Autodesk Fusion 360 part; units mm, degrees
(part 7 of 7)
  line L506 (59.905, -71.6419) -> (59.8713, -71.7229)
  line L507 (59.8713, -71.7229) -> (59.8391, -71.8051)
  line L508 (59.8391, -71.8051) -> (59.9395, -71.9042)
  line L509 (59.9395, -71.9042) -> (60.0412, -72.002)
  line L510 (60.0412, -72.002) -> (60.1441, -72.0986)
  line L511 (60.1441, -72.0986) -> (60.225, -72.0631)
  line L512 (60.225, -72.0631) -> (60.3047, -72.0264)
  line L513 (60.3047, -72.0264) -> (60.3829, -71.9882)
  line L514 (60.3829, -71.9882) -> (60.4597, -71.9486)
  line L515 (60.4597, -71.9486) -> (60.535, -71.9075)
  line L516 (60.535, -71.9075) -> (60.6087, -71.8648)
  line L517 (60.6087, -71.8648) -> (60.6807, -71.8206)
  line L518 (60.6807, -71.8206) -> (60.7508, -71.7746)
  line L519 (60.7508, -71.7746) -> (60.8189, -71.7268)
  line L520 (60.8189, -71.7268) -> (60.8846, -71.6768)
  line L521 (60.8846, -71.6768) -> (60.9474, -71.6243)
  line L522 (60.9474, -71.6243) -> (61.006, -71.568)
  line L523 (61.006, -71.568) -> (61.2294, -71.3134)
  line L524 (61.2294, -71.3134) -> (61.3835, -71.4459)
  line L525 (61.3835, -71.4459) -> (61.5404, -71.5752)
  line L526 (61.5404, -71.5752) -> (61.7, -71.7012)
  line L527 (61.7, -71.7012) -> (61.8621, -71.8238)
  line L528 (61.8621, -71.8238) -> (61.6605, -72.096)
  line L529 (61.6605, -72.096) -> (61.6179, -72.1651)
  line L530 (61.6179, -72.1651) -> (61.5798, -72.2377)
  line L531 (61.5798, -72.2377) -> (61.5449, -72.3125)
  line L532 (61.5449, -72.3125) -> (61.5125, -72.3891)
  line L533 (61.5125, -72.3891) -> (61.4824, -72.4674)
  line L534 (61.4824, -72.4674) -> (61.4544, -72.5471)
  line L535 (61.4544, -72.5471) -> (61.4283, -72.6281)
  line L536 (61.4283, -72.6281) -> (61.4041, -72.7104)
  line L537 (61.4041, -72.7104) -> (61.3816, -72.7939)
  line L538 (61.3816, -72.7939) -> (61.3609, -72.8784)
  line L539 (61.3609, -72.8784) -> (61.3418, -72.964)
  line L540 (61.3418, -72.964) -> (61.3242, -73.0507)
  line L541 (61.3242, -73.0507) -> (61.4404, -73.1308)
  line L542 (61.4404, -73.1308) -> (61.5575, -73.2095)
  line L543 (61.5575, -73.2095) -> (61.6756, -73.2867)
  line L544 (61.6756, -73.2867) -> (61.7492, -73.2378)
  line L545 (61.7492, -73.2378) -> (61.8212, -73.1877)
  line L546 (61.8212, -73.1877) -> (61.8916, -73.1365)
  line L547 (61.8916, -73.1365) -> (61.9604, -73.0841)
  line L548 (61.9604, -73.0841) -> (62.0274, -73.0306)
  line L549 (62.0274, -73.0306) -> (62.0926, -72.9758)
  line L550 (62.0926, -72.9758) -> (62.1558, -72.9198)
  line L551 (62.1558, -72.9198) -> (62.2169, -72.8623)
  line L552 (62.2169, -72.8623) -> (62.2756, -72.8034)
  line L553 (62.2756, -72.8034) -> (62.3316, -72.7427)
  line L554 (62.3316, -72.7427) -> (62.3844, -72.6801)
  line L555 (62.3844, -72.6801) -> (62.4323, -72.6145)
  line L556 (62.4323, -72.6145) -> (62.608, -72.325)
  line L557 (62.608, -72.325) -> (62.7829, -72.4287)
  line L558 (62.7829, -72.4287) -> (62.9599, -72.5288)
  line L559 (62.9599, -72.5288) -> (63.1388, -72.6252)
  line L560 (63.1388, -72.6252) -> (63.3198, -72.7178)
  line L561 (63.3198, -72.7178) -> (63.1686, -73.0209)
  line L562 (63.1686, -73.0209) -> (63.1386, -73.0963)
  line L563 (63.1386, -73.0963) -> (63.1137, -73.1744)
  line L564 (63.1137, -73.1744) -> (63.0923, -73.2541)
  line L565 (63.0923, -73.2541) -> (63.0737, -73.3352)
  line L566 (63.0737, -73.3352) -> (63.0577, -73.4175)
  line L567 (63.0577, -73.4175) -> (63.0439, -73.5009)
  line L568 (63.0439, -73.5009) -> (63.0323, -73.5852)
  line L569 (63.0323, -73.5852) -> (63.0227, -73.6704)
  line L570 (63.0227, -73.6704) -> (63.0151, -73.7565)
  line L571 (63.0151, -73.7565) -> (63.0093, -73.8434)
  line L572 (63.0093, -73.8434) -> (63.0054, -73.9311)
  line L573 (63.0054, -73.9311) -> (63.0032, -74.0194)
  line L574 (63.0032, -74.0194) -> (63.1314, -74.0782)
  line L575 (63.1314, -74.0782) -> (63.2604, -74.1353)
  line L576 (63.2604, -74.1353) -> (63.3901, -74.1908)
  line L577 (63.3901, -74.1908) -> (63.4541, -74.1299)
  line L578 (63.4541, -74.1299) -> (63.5163, -74.068)
  line L579 (63.5163, -74.068) -> (63.5768, -74.0054)
  line L580 (63.5768, -74.0054) -> (63.6355, -73.9419)
  line L581 (63.6355, -73.9419) -> (63.6922, -73.8775)
  line L582 (63.6922, -73.8775) -> (63.7468, -73.8123)
  line L583 (63.7468, -73.8123) -> (63.7993, -73.7461)
  line L584 (63.7993, -73.7461) -> (63.8495, -73.6789)
  line L585 (63.8495, -73.6789) -> (63.8971, -73.6106)
  line L586 (63.8971, -73.6106) -> (63.9418, -73.5412)
  line L587 (63.9418, -73.5412) -> (63.9829, -73.4704)
  line L588 (63.9829, -73.4704) -> (64.0186, -73.3974)
  line L589 (64.0186, -73.3974) -> (64.1414, -73.0818)
  line L590 (64.1414, -73.0818) -> (64.3316, -73.1536)
  line L591 (64.3316, -73.1536) -> (64.5233, -73.2214)
  line L592 (64.5233, -73.2214) -> (64.7163, -73.2852)
  line L593 (64.7163, -73.2852) -> (64.9106, -73.3451)
  line L594 (64.9106, -73.3451) -> (64.8143, -73.6698)
  line L595 (64.8143, -73.6698) -> (64.7978, -73.7493)
  line L596 (64.7978, -73.7493) -> (64.7869, -73.8305)
  line L597 (64.7869, -73.8305) -> (64.7797, -73.9127)
  line L598 (64.7797, -73.9127) -> (64.7755, -73.9958)
  line L599 (64.7755, -73.9958) -> (64.7739, -74.0796)
  line L600 (64.7739, -74.0796) -> (64.7749, -74.1641)
  line L601 (64.7749, -74.1641) -> (64.7781, -74.2492)
  line L602 (64.7781, -74.2492) -> (64.7835, -74.3348)
  line L603 (64.7835, -74.3348) -> (64.7909, -74.4209)
  line L604 (64.7909, -74.4209) -> (64.8003, -74.5075)
  line L605 (64.8003, -74.5075) -> (64.8116, -74.5945)
  line L606 (64.8116, -74.5945) -> (64.8248, -74.6819)
  line L607 (64.8248, -74.6819) -> (64.9613, -74.7175)
  line L608 (64.9613, -74.7175) -> (65.0983, -74.7514)
  line L609 (65.0983, -74.7514) -> (65.2357, -74.7835)
  line L610 (65.2357, -74.7835) -> (65.2881, -74.7123)
  line L611 (65.2881, -74.7123) -> (65.3386, -74.6407)
  line L612 (65.3386, -74.6407) -> (65.3873, -74.5685)
  line L613 (65.3873, -74.5685) -> (65.434, -74.4957)
  line L614 (65.434, -74.4957) -> (65.4787, -74.4225)
  line L615 (65.4787, -74.4225) -> (65.5212, -74.3487)
  line L616 (65.5212, -74.3487) -> (65.5614, -74.2744)
  line L617 (65.5614, -74.2744) -> (65.5991, -74.1996)
  line L618 (65.5991, -74.1996) -> (65.6342, -74.1241)
  line L619 (65.6342, -74.1241) -> (65.6661, -74.048)
  line L620 (65.6661, -74.048) -> (65.6943, -73.9711)
  line L621 (65.6943, -73.9711) -> (65.7168, -73.893)
  line L622 (65.7168, -73.893) -> (65.783, -73.5609)
  line L623 (65.783, -73.5609) -> (65.9827, -73.5985)
  line L624 (65.9827, -73.5985) -> (66.1833, -73.632)
  line L625 (66.1833, -73.632) -> (66.3844, -73.6614)
  line L626 (66.3844, -73.6614) -> (66.5861, -73.6866)
  line L627 (66.5861, -73.6866) -> (66.5477, -74.023)
  line L628 (66.5477, -74.023) -> (66.5453, -74.1042)
  line L629 (66.5453, -74.1042) -> (66.5486, -74.1861)
  line L630 (66.5486, -74.1861) -> (66.5558, -74.2683)
  line L631 (66.5558, -74.2683) -> (66.5661, -74.3509)
  line L632 (66.5661, -74.3509) -> (66.5791, -74.4337)
  line L633 (66.5791, -74.4337) -> (66.5947, -74.5167)
  line L634 (66.5947, -74.5167) -> (66.6126, -74.6)
  line L635 (66.6126, -74.6) -> (66.6328, -74.6834)
  line L636 (66.6328, -74.6834) -> (66.6551, -74.7669)
  line L637 (66.6551, -74.7669) -> (66.6794, -74.8505)
  line L638 (66.6794, -74.8505) -> (66.7056, -74.9342)
  line L639 (66.7056, -74.9342) -> (66.7338, -75.0179)
  line L640 (66.7338, -75.0179) -> (66.8744, -75.0293)
  line L641 (66.8744, -75.0293) -> (67.0152, -75.0389)
  line L642 (67.0152, -75.0389) -> (67.1561, -75.0467)
  line L643 (67.1561, -75.0467) -> (67.1953, -74.9675)
  line L644 (67.1953, -74.9675) -> (67.2326, -74.8881)
  line L645 (67.2326, -74.8881) -> (67.268, -74.8086)
  line L646 (67.268, -74.8086) -> (67.3014, -74.7289)
  line L647 (67.3014, -74.7289) -> (67.3327, -74.649)
  line L648 (67.3327, -74.649) -> (67.3618, -74.569)
  line L649 (67.3618, -74.569) -> (67.3884, -74.4888)
  line L650 (67.3884, -74.4888) -> (67.4126, -74.4085)
  line L651 (67.4126, -74.4085) -> (67.434, -74.3281)
  line L652 (67.434, -74.3281) -> (67.4522, -74.2476)
  line L653 (67.4522, -74.2476) -> (67.4666, -74.167)
  line L654 (67.4666, -74.167) -> (67.4752, -74.0862)
  line L655 (67.4752, -74.0862) -> (67.4827, -73.7476)
  line L656 (67.4827, -73.7476) -> (67.686, -73.75)
  line L657 (67.686, -73.75) -> (67.8893, -73.7482)
  line L658 (67.8893, -73.7482) -> (68.0925, -73.7421)
  line L659 (68.0925, -73.7421) -> (68.2955, -73.7319)
  line L660 (68.2955, -73.7319) -> (68.3161, -74.07)
  line L661 (68.3161, -74.07) -> (68.3278, -74.1503)
  line L662 (68.3278, -74.1503) -> (68.3453, -74.2304)
  line L663 (68.3453, -74.2304) -> (68.3666, -74.3101)
  line L664 (68.3666, -74.3101) -> (68.3911, -74.3896)
  line L665 (68.3911, -74.3896) -> (68.4184, -74.4689)
  line L666 (68.4184, -74.4689) -> (68.4481, -74.548)
  line L667 (68.4481, -74.548) -> (68.4803, -74.6268)
  line L668 (68.4803, -74.6268) -> (68.5146, -74.7055)
  line L669 (68.5146, -74.7055) -> (68.551, -74.7838)
  line L670 (68.551, -74.7838) -> (68.5895, -74.862)
  line L671 (68.5895, -74.862) -> (68.6298, -74.9398)
  line L672 (68.6298, -74.9398) -> (68.6721, -75.0174)
  line L673 (68.6721, -75.0174) -> (68.8126, -75.0042)
  line L674 (68.8126, -75.0042) -> (68.9529, -74.9892)
  line L675 (68.9529, -74.9892) -> (69.093, -74.9724)
  line L676 (69.093, -74.9724) -> (69.1179, -74.8876)
  line L677 (69.1179, -74.8876) -> (69.1409, -74.803)
  line L678 (69.1409, -74.803) -> (69.1619, -74.7185)
  line L679 (69.1619, -74.7185) -> (69.181, -74.6342)
  line L680 (69.181, -74.6342) -> (69.1979, -74.5501)
  line L681 (69.1979, -74.5501) -> (69.2126, -74.4662)
  line L682 (69.2126, -74.4662) -> (69.225, -74.3826)
  line L683 (69.225, -74.3826) -> (69.2348, -74.2994)
  line L684 (69.2348, -74.2994) -> (69.2419, -74.2165)
  line L685 (69.2419, -74.2165) -> (69.2459, -74.134)
  line L686 (69.2459, -74.134) -> (69.246, -74.0521)
  line L687 (69.246, -74.0521) -> (69.2405, -73.9711)
  line L688 (69.2405, -73.9711) -> (69.1891, -73.6363)
  line L689 (69.1891, -73.6363) -> (69.3897, -73.6034)
  line L690 (69.3897, -73.6034) -> (69.5896, -73.5663)
  line L691 (69.5896, -73.5663) -> (69.7887, -73.5251)
  line L692 (69.7887, -73.5251) -> (69.9868, -73.4797)
  line L693 (69.9868, -73.4797) -> (70.0658, -73.8091)
  line L694 (70.0658, -73.8091) -> (70.0913, -73.8862)
  line L695 (70.0913, -73.8862) -> (70.1224, -73.962)
  line L696 (70.1224, -73.962) -> (70.1573, -74.0368)
  line L697 (70.1573, -74.0368) -> (70.1952, -74.1109)
  line L698 (70.1952, -74.1109) -> (70.2358, -74.1842)
  line L699 (70.2358, -74.1842) -> (70.2788, -74.2569)
  line L700 (70.2788, -74.2569) -> (70.3241, -74.329)
  line L701 (70.3241, -74.329) -> (70.3716, -74.4005)
  line L702 (70.3716, -74.4005) -> (70.4211, -74.4713)
  line L703 (70.4211, -74.4713) -> (70.4725, -74.5416)
  line L704 (70.4725, -74.5416) -> (70.5258, -74.6112)
  line L705 (70.5258, -74.6112) -> (70.5809, -74.6803)
  line L706 (70.5809, -74.6803) -> (70.717, -74.6429)
  line L707 (70.717, -74.6429) -> (70.8525, -74.6038)
  line L708 (70.8525, -74.6038) -> (70.9876, -74.5629)
  line L709 (70.9876, -74.5629) -> (70.9974, -74.4751)
  line L710 (70.9974, -74.4751) -> (71.0053, -74.3877)
  line L711 (71.0053, -74.3877) -> (71.0114, -74.3009)
  line L712 (71.0114, -74.3009) -> (71.0155, -74.2145)
  line L713 (71.0155, -74.2145) -> (71.0175, -74.1288)
  line L714 (71.0175, -74.1288) -> (71.0175, -74.0436)
  line L715 (71.0175, -74.0436) -> (71.0151, -73.9592)
  line L716 (71.0151, -73.9592) -> (71.0104, -73.8755)
  line L717 (71.0104, -73.8755) -> (71.003, -73.7926)
  line L718 (71.003, -73.7926) -> (70.9926, -73.7107)
  line L719 (70.9926, -73.7107) -> (70.9785, -73.63)
  line L720 (70.9785, -73.63) -> (70.959, -73.5512)
  line L721 (70.959, -73.5512) -> (70.8502, -73.2304)
  line L722 (70.8502, -73.2304) -> (71.0421, -73.1632)
  line L723 (71.0421, -73.1632) -> (71.2325, -73.0919)
  line L724 (71.2325, -73.0919) -> (71.4214, -73.0168)
  line L725 (71.4214, -73.0168) -> (71.6087, -72.9377)
  line L726 (71.6087, -72.9377) -> (71.7436, -73.2483)
  line L727 (71.7436, -73.2483) -> (71.7821, -73.3198)
  line L728 (71.7821, -73.3198) -> (71.8259, -73.389)
  line L729 (71.8259, -73.389) -> (71.8732, -73.4567)
  line L730 (71.8732, -73.4567) -> (71.9234, -73.5231)
  line L731 (71.9234, -73.5231) -> (71.9761, -73.5883)
  line L732 (71.9761, -73.5883) -> (72.0312, -73.6524)
  line L733 (72.0312, -73.6524) -> (72.0883, -73.7155)
  line L734 (72.0883, -73.7155) -> (72.1475, -73.7776)
  line L735 (72.1475, -73.7776) -> (72.2085, -73.8388)
  line L736 (72.2085, -73.8388) -> (72.2713, -73.8991)
  line L737 (72.2713, -73.8991) -> (72.3359, -73.9584)
  line L738 (72.3359, -73.9584) -> (72.4022, -74.0169)
  line L739 (72.4022, -74.0169) -> (72.5297, -73.9564)
  line L740 (72.5297, -73.9564) -> (72.6564, -73.8943)
  line L741 (72.6564, -73.8943) -> (72.7823, -73.8306)
  line L742 (72.7823, -73.8306) -> (72.7767, -73.7425)
  line L743 (72.7767, -73.7425) -> (72.7693, -73.655)
  line L744 (72.7693, -73.655) -> (72.7602, -73.5685)
  line L745 (72.7602, -73.5685) -> (72.7493, -73.4827)
  line L746 (72.7493, -73.4827) -> (72.7364, -73.3979)
  line L747 (72.7364, -73.3979) -> (72.7215, -73.3141)
  line L748 (72.7215, -73.3141) -> (72.7046, -73.2313)
  line L749 (72.7046, -73.2313) -> (72.6854, -73.1497)
  line L750 (72.6854, -73.1497) -> (72.6637, -73.0694)
  line L751 (72.6637, -73.0694) -> (72.6392, -72.9905)
  line L752 (72.6392, -72.9905) -> (72.6114, -72.9135)
  line L753 (72.6114, -72.9135) -> (72.5784, -72.8392)
  line L754 (72.5784, -72.8392) -> (72.4156, -72.5423)
  line L755 (72.4156, -72.5423) -> (72.5929, -72.4427)
  line L756 (72.5929, -72.4427) -> (72.768, -72.3395)
  line L757 (72.768, -72.3395) -> (72.941, -72.2327)
  line L758 (72.941, -72.2327) -> (73.1117, -72.1223)
  line L759 (73.1117, -72.1223) -> (73.2985, -72.4048)
  line L760 (73.2985, -72.4048) -> (73.3489, -72.4685)
  line L761 (73.3489, -72.4685) -> (73.4041, -72.529)
  line L762 (73.4041, -72.529) -> (73.4624, -72.5874)
  line L763 (73.4624, -72.5874) -> (73.5233, -72.6441)
  line L764 (73.5233, -72.6441) -> (73.5866, -72.6991)
  line L765 (73.5866, -72.6991) -> (73.6519, -72.7527)
  line L766 (73.6519, -72.7527) -> (73.7191, -72.8049)
  line L767 (73.7191, -72.8049) -> (73.7882, -72.8559)
  line L768 (73.7882, -72.8559) -> (73.8589, -72.9055)
  line L769 (73.8589, -72.9055) -> (73.9313, -72.954)
  line L770 (73.9313, -72.954) -> (74.0052, -73.0012)
  line L771 (74.0052, -73.0012) -> (74.0806, -73.0473)
  line L772 (74.0806, -73.0473) -> (74.1956, -72.9656)
  line L773 (74.1956, -72.9656) -> (74.3096, -72.8824)
  line L774 (74.3096, -72.8824) -> (74.4226, -72.7979)
  line L775 (74.4226, -72.7979) -> (74.4017, -72.712)
  line L776 (74.4017, -72.712) -> (74.3793, -72.6272)
  line L777 (74.3793, -72.6272) -> (74.3553, -72.5435)
  line L778 (74.3553, -72.5435) -> (74.3296, -72.4609)
  line L779 (74.3296, -72.4609) -> (74.3022, -72.3797)
  line L780 (74.3022, -72.3797) -> (74.273, -72.2997)
  line L781 (74.273, -72.2997) -> (74.242, -72.2211)
  line L782 (74.242, -72.2211) -> (74.2089, -72.1441)
  line L783 (74.2089, -72.1441) -> (74.1736, -72.0687)
  line L784 (74.1736, -72.0687) -> (74.1358, -71.9953)
  line L785 (74.1358, -71.9953) -> (74.095, -71.9243)
  line L786 (74.095, -71.9243) -> (74.0497, -71.8569)
  line L787 (74.0497, -71.8569) -> (73.8378, -71.5927)
  line L788 (73.8378, -71.5927) -> (73.995, -71.4639)
  line L789 (73.995, -71.4639) -> (74.1496, -71.3318)
  line L790 (74.1496, -71.3318) -> (74.3014, -71.1966)
  line L791 (74.3014, -71.1966) -> (74.4503, -71.0582)
  line L792 (74.4503, -71.0582) -> (74.6834, -71.304)
  line L793 (74.6834, -71.304) -> (74.744, -71.358)
  line L794 (74.744, -71.358) -> (74.8089, -71.4081)
  line L795 (74.8089, -71.4081) -> (74.8765, -71.4554)
  line L796 (74.8765, -71.4554) -> (74.9463, -71.5006)
  line L797 (74.9463, -71.5006) -> (75.0182, -71.5439)
  line L798 (75.0182, -71.5439) -> (75.0918, -71.5853)
  line L799 (75.0918, -71.5853) -> (75.1671, -71.6251)
  line L800 (75.1671, -71.6251) -> (75.2439, -71.6632)
  line L801 (75.2439, -71.6632) -> (75.3222, -71.6998)
  line L802 (75.3222, -71.6998) -> (75.4019, -71.735)
  line L803 (75.4019, -71.735) -> (75.4829, -71.7687)
  line L804 (75.4829, -71.7687) -> (75.5651, -71.8009)
  line L805 (75.5651, -71.8009) -> (75.6642, -71.7005)
  line L806 (75.6642, -71.7005) -> (75.762, -71.5988)
  line L807 (75.762, -71.5988) -> (75.8586, -71.4959)
  line L808 (75.8586, -71.4959) -> (75.8231, -71.415)
  line L809 (75.8231, -71.415) -> (75.7864, -71.3353)
  line L810 (75.7864, -71.3353) -> (75.7482, -71.2571)
  line L811 (75.7482, -71.2571) -> (75.7086, -71.1803)
  line L812 (75.7086, -71.1803) -> (75.6675, -71.105)
  line L813 (75.6675, -71.105) -> (75.6248, -71.0313)
  line L814 (75.6248, -71.0313) -> (75.5806, -70.9593)
  line L815 (75.5806, -70.9593) -> (75.5346, -70.8892)
  line L816 (75.5346, -70.8892) -> (75.4868, -70.8211)
  line L817 (75.4868, -70.8211) -> (75.4368, -70.7554)
  line L818 (75.4368, -70.7554) -> (75.3843, -70.6926)
  line L819 (75.3843, -70.6926) -> (75.328, -70.634)
  line L820 (75.328, -70.634) -> (75.0734, -70.4106)
  line L821 (75.0734, -70.4106) -> (75.2059, -70.2565)
  line L822 (75.2059, -70.2565) -> (75.3352, -70.0996)
  line L823 (75.3352, -70.0996) -> (75.4612, -69.94)
  line L824 (75.4612, -69.94) -> (75.5838, -69.7779)
  line L825 (75.5838, -69.7779) -> (75.856, -69.9795)
  line L826 (75.856, -69.9795) -> (75.9251, -70.0221)
  line L827 (75.9251, -70.0221) -> (75.9977, -70.0602)
  line L828 (75.9977, -70.0602) -> (76.0725, -70.0951)
  line L829 (76.0725, -70.0951) -> (76.1491, -70.1275)
  line L830 (76.1491, -70.1275) -> (76.2274, -70.1576)
  line L831 (76.2274, -70.1576) -> (76.3071, -70.1856)
  line L832 (76.3071, -70.1856) -> (76.3881, -70.2117)
  line L833 (76.3881, -70.2117) -> (76.4704, -70.2359)
  line L834 (76.4704, -70.2359) -> (76.5539, -70.2584)
  line L835 (76.5539, -70.2584) -> (76.6384, -70.2791)
  line L836 (76.6384, -70.2791) -> (76.724, -70.2982)
  line L837 (76.724, -70.2982) -> (76.8107, -70.3158)
  line L838 (76.8107, -70.3158) -> (76.8908, -70.1996)
  line L839 (76.8908, -70.1996) -> (76.9695, -70.0825)
  line L840 (76.9695, -70.0825) -> (77.0467, -69.9644)
  line L841 (77.0467, -69.9644) -> (76.9978, -69.8908)
  line L842 (76.9978, -69.8908) -> (76.9477, -69.8188)
  line L843 (76.9477, -69.8188) -> (76.8965, -69.7484)
  line L844 (76.8965, -69.7484) -> (76.8441, -69.6796)
  line L845 (76.8441, -69.6796) -> (76.7906, -69.6126)
  line L846 (76.7906, -69.6126) -> (76.7358, -69.5474)
  line L847 (76.7358, -69.5474) -> (76.6798, -69.4842)
  line L848 (76.6798, -69.4842) -> (76.6223, -69.4231)
  line L849 (76.6223, -69.4231) -> (76.5634, -69.3644)
  line L850 (76.5634, -69.3644) -> (76.5027, -69.3084)
  line L851 (76.5027, -69.3084) -> (76.4401, -69.2556)
  line L852 (76.4401, -69.2556) -> (76.3745, -69.2077)
  line L853 (76.3745, -69.2077) -> (76.085, -69.032)
  line L854 (76.085, -69.032) -> (76.1887, -68.8571)
  line L855 (76.1887, -68.8571) -> (76.2888, -68.6801)
  line L856 (76.2888, -68.6801) -> (76.3852, -68.5012)
  line L857 (76.3852, -68.5012) -> (76.4778, -68.3202)
  line L858 (76.4778, -68.3202) -> (76.7809, -68.4714)
  line L859 (76.7809, -68.4714) -> (76.8563, -68.5014)
  line L860 (76.8563, -68.5014) -> (76.9344, -68.5263)
  line L861 (76.9344, -68.5263) -> (77.0141, -68.5477)
  line L862 (77.0141, -68.5477) -> (77.0952, -68.5663)
  line L863 (77.0952, -68.5663) -> (77.1775, -68.5823)
  line L864 (77.1775, -68.5823) -> (77.2609, -68.5961)
  line L865 (77.2609, -68.5961) -> (77.3452, -68.6077)
  line L866 (77.3452, -68.6077) -> (77.4304, -68.6173)
  line L867 (77.4304, -68.6173) -> (77.5165, -68.6249)
  line L868 (77.5165, -68.6249) -> (77.6034, -68.6307)
  line L869 (77.6034, -68.6307) -> (77.6911, -68.6346)
  line L870 (77.6911, -68.6346) -> (77.7794, -68.6368)
  line L871 (77.7794, -68.6368) -> (77.8382, -68.5086)
  line L872 (77.8382, -68.5086) -> (77.8953, -68.3796)
  line L873 (77.8953, -68.3796) -> (77.9508, -68.2499)
  line L874 (77.9508, -68.2499) -> (77.8899, -68.1859)
  line L875 (77.8899, -68.1859) -> (77.828, -68.1237)
  line L876 (77.828, -68.1237) -> (77.7654, -68.0632)
  line L877 (77.7654, -68.0632) -> (77.7019, -68.0045)
  line L878 (77.7019, -68.0045) -> (77.6375, -67.9478)
  line L879 (77.6375, -67.9478) -> (77.5723, -67.8932)
  line L880 (77.5723, -67.8932) -> (77.5061, -67.8407)
  line L881 (77.5061, -67.8407) -> (77.4389, -67.7905)
  line L882 (77.4389, -67.7905) -> (77.3706, -67.7429)
  line L883 (77.3706, -67.7429) -> (77.3012, -67.6982)
  line L884 (77.3012, -67.6982) -> (77.2304, -67.6571)
  line L885 (77.2304, -67.6571) -> (77.1574, -67.6214)
  line L886 (77.1574, -67.6214) -> (76.8418, -67.4986)
  line L887 (76.8418, -67.4986) -> (76.9136, -67.3084)
  line L888 (76.9136, -67.3084) -> (76.9814, -67.1167)
  line L889 (76.9814, -67.1167) -> (77.0452, -66.9237)
  line L890 (77.0452, -66.9237) -> (77.1051, -66.7294)
  line L891 (77.1051, -66.7294) -> (77.4298, -66.8257)
  line L892 (77.4298, -66.8257) -> (77.5093, -66.8422)
  line L893 (77.5093, -66.8422) -> (77.5905, -66.8531)
  line L894 (77.5905, -66.8531) -> (77.6727, -66.8603)
  line L895 (77.6727, -66.8603) -> (77.7558, -66.8645)
  line L896 (77.7558, -66.8645) -> (77.8396, -66.8661)
  line L897 (77.8396, -66.8661) -> (77.9241, -66.8651)
  line L898 (77.9241, -66.8651) -> (78.0092, -66.8619)
  line L899 (78.0092, -66.8619) -> (78.0948, -66.8565)
  line L900 (78.0948, -66.8565) -> (78.1809, -66.8491)
  line L901 (78.1809, -66.8491) -> (78.2675, -66.8397)
  line L902 (78.2675, -66.8397) -> (78.3545, -66.8284)
  line L903 (78.3545, -66.8284) -> (78.4419, -66.8152)
  line L904 (78.4419, -66.8152) -> (78.4775, -66.6787)
  line L905 (78.4775, -66.6787) -> (78.5114, -66.5417)
  line L906 (78.5114, -66.5417) -> (78.5435, -66.4043)
  line L907 (78.5435, -66.4043) -> (78.4723, -66.3519)
  line L908 (78.4723, -66.3519) -> (78.4007, -66.3014)
  line L909 (78.4007, -66.3014) -> (78.3285, -66.2527)
  line L910 (78.3285, -66.2527) -> (78.2557, -66.206)
  line L911 (78.2557, -66.206) -> (78.1825, -66.1613)
  line L912 (78.1825, -66.1613) -> (78.1087, -66.1188)
  line L913 (78.1087, -66.1188) -> (78.0344, -66.0786)
  line L914 (78.0344, -66.0786) -> (77.9596, -66.0409)
  line L915 (77.9596, -66.0409) -> (77.8841, -66.0058)
  line L916 (77.8841, -66.0058) -> (77.808, -65.9739)
  line L917 (77.808, -65.9739) -> (77.7311, -65.9457)
  line L918 (77.7311, -65.9457) -> (77.653, -65.9232)
  line L919 (77.653, -65.9232) -> (77.3209, -65.857)
  line L920 (77.3209, -65.857) -> (77.3585, -65.6573)
  line L921 (77.3585, -65.6573) -> (77.392, -65.4567)
  line L922 (77.392, -65.4567) -> (77.4214, -65.2556)
  line L923 (77.4214, -65.2556) -> (77.4466, -65.0539)
  line L924 (77.4466, -65.0539) -> (77.783, -65.0923)
  line L925 (77.783, -65.0923) -> (77.8642, -65.0947)
  line L926 (77.8642, -65.0947) -> (77.9461, -65.0914)
  line L927 (77.9461, -65.0914) -> (78.0283, -65.0842)
  line L928 (78.0283, -65.0842) -> (78.1109, -65.0739)
  line L929 (78.1109, -65.0739) -> (78.1937, -65.0609)
  line L930 (78.1937, -65.0609) -> (78.2767, -65.0453)
  line L931 (78.2767, -65.0453) -> (78.36, -65.0274)
  line L932 (78.36, -65.0274) -> (78.4434, -65.0072)
  line L933 (78.4434, -65.0072) -> (78.5269, -64.9849)
  line L934 (78.5269, -64.9849) -> (78.6105, -64.9606)
  line L935 (78.6105, -64.9606) -> (78.6942, -64.9344)
  line L936 (78.6942, -64.9344) -> (78.7779, -64.9062)
  line L937 (78.7779, -64.9062) -> (78.7893, -64.7656)
  line L938 (78.7893, -64.7656) -> (78.7989, -64.6248)
  line L939 (78.7989, -64.6248) -> (78.8067, -64.4839)
  line L940 (78.8067, -64.4839) -> (78.7275, -64.4447)
  line L941 (78.7275, -64.4447) -> (78.6481, -64.4074)
  line L942 (78.6481, -64.4074) -> (78.5686, -64.372)
  line L943 (78.5686, -64.372) -> (78.4889, -64.3386)
  line L944 (78.4889, -64.3386) -> (78.409, -64.3073)
  line L945 (78.409, -64.3073) -> (78.329, -64.2782)
  line L946 (78.329, -64.2782) -> (78.2488, -64.2516)
  line L947 (78.2488, -64.2516) -> (78.1685, -64.2274)
  line L948 (78.1685, -64.2274) -> (78.0881, -64.206)
  line L949 (78.0881, -64.206) -> (78.0076, -64.1878)
  line L950 (78.0076, -64.1878) -> (77.927, -64.1734)
  line L951 (77.927, -64.1734) -> (77.8462, -64.1648)
  line L952 (77.8462, -64.1648) -> (77.5076, -64.1573)
  line L953 (77.5076, -64.1573) -> (77.51, -63.954)
  line L954 (77.51, -63.954) -> (77.5082, -63.7507)
  line L955 (77.5082, -63.7507) -> (77.5021, -63.5475)
  line L956 (77.5021, -63.5475) -> (77.4919, -63.3445)
  line L957 (77.4919, -63.3445) -> (77.83, -63.3239)
  line L958 (77.83, -63.3239) -> (77.9103, -63.3122)
  line L959 (77.9103, -63.3122) -> (77.9904, -63.2947)
  line L960 (77.9904, -63.2947) -> (78.0701, -63.2734)
  line L961 (78.0701, -63.2734) -> (78.1496, -63.2489)
  line L962 (78.1496, -63.2489) -> (78.2289, -63.2216)
  line L963 (78.2289, -63.2216) -> (78.308, -63.1919)
  line L964 (78.308, -63.1919) -> (78.3868, -63.1597)
  line L965 (78.3868, -63.1597) -> (78.4655, -63.1254)
  line L966 (78.4655, -63.1254) -> (78.5438, -63.089)
  line L967 (78.5438, -63.089) -> (78.622, -63.0505)
  line L968 (78.622, -63.0505) -> (78.6998, -63.0102)
  line L969 (78.6998, -63.0102) -> (78.7774, -62.9679)
  line L970 (78.7774, -62.9679) -> (78.7642, -62.8274)
  line L971 (78.7642, -62.8274) -> (78.7492, -62.6871)
  line L972 (78.7492, -62.6871) -> (78.7324, -62.547)
  line L973 (78.7324, -62.547) -> (78.6476, -62.5221)
  line L974 (78.6476, -62.5221) -> (78.563, -62.4991)
  line L975 (78.563, -62.4991) -> (78.4785, -62.4781)
  line L976 (78.4785, -62.4781) -> (78.3942, -62.459)
  line L977 (78.3942, -62.459) -> (78.3101, -62.4421)
  line L978 (78.3101, -62.4421) -> (78.2262, -62.4274)
  line L979 (78.2262, -62.4274) -> (78.1426, -62.415)
  line L980 (78.1426, -62.415) -> (78.0594, -62.4052)
  line L981 (78.0594, -62.4052) -> (77.9765, -62.3981)
  line L982 (77.9765, -62.3981) -> (77.894, -62.3941)
  line L983 (77.894, -62.3941) -> (77.8121, -62.394)
  line L984 (77.8121, -62.394) -> (77.7311, -62.3995)
  line L985 (77.7311, -62.3995) -> (77.3963, -62.4509)
  line L986 (77.3963, -62.4509) -> (77.3634, -62.2503)
  line L987 (77.3634, -62.2503) -> (77.3263, -62.0504)
  line L988 (77.3263, -62.0504) -> (77.2851, -61.8513)
  line L989 (77.2851, -61.8513) -> (77.2397, -61.6532)
  line L990 (77.2397, -61.6532) -> (77.5691, -61.5742)
  line L991 (77.5691, -61.5742) -> (77.6462, -61.5487)
  line L992 (77.6462, -61.5487) -> (77.722, -61.5176)
  line L993 (77.722, -61.5176) -> (77.7968, -61.4827)
  line L994 (77.7968, -61.4827) -> (77.8709, -61.4448)
  line L995 (77.8709, -61.4448) -> (77.9442, -61.4042)
  line L996 (77.9442, -61.4042) -> (78.0169, -61.3612)
  line L997 (78.0169, -61.3612) -> (78.089, -61.3159)
  line L998 (78.089, -61.3159) -> (78.1605, -61.2684)
  line L999 (78.1605, -61.2684) -> (78.2313, -61.2189)
  line L1000 (78.2313, -61.2189) -> (78.3016, -61.1675)
  line L1001 (78.3016, -61.1675) -> (78.3712, -61.1142)
  line L1002 (78.3712, -61.1142) -> (78.4403, -61.0591)
  line L1003 (78.4403, -61.0591) -> (78.4029, -60.923)
  line L1004 (78.4029, -60.923) -> (78.3638, -60.7875)
  line L1005 (78.3638, -60.7875) -> (78.3229, -60.6524)
  line L1006 (78.3229, -60.6524) -> (78.2351, -60.6426)
  line L1007 (78.2351, -60.6426) -> (78.1477, -60.6347)
  line L1008 (78.1477, -60.6347) -> (78.0609, -60.6286)
  line L1009 (78.0609, -60.6286) -> (77.9745, -60.6245)
  line L1010 (77.9745, -60.6245) -> (77.8888, -60.6225)
  line L1011 (77.8888, -60.6225) -> (77.8036, -60.6225)
  line L1012 (77.8036, -60.6225) -> (77.7192, -60.6249)
  line L1013 (77.7192, -60.6249) -> (77.6355, -60.6296)
  line L1014 (77.6355, -60.6296) -> (77.5526, -60.637)
  line L1015 (77.5526, -60.637) -> (77.4707, -60.6474)
  line L1016 (77.4707, -60.6474) -> (77.39, -60.6615)
  line L1017 (77.39, -60.6615) -> (77.3112, -60.681)
  line L1018 (77.3112, -60.681) -> (76.9904, -60.7898)
  line L1019 (76.9904, -60.7898) -> (76.9232, -60.5979)
  line L1020 (76.9232, -60.5979) -> (76.8519, -60.4075)
  line L1021 (76.8519, -60.4075) -> (76.7768, -60.2186)
  line L1022 (76.7768, -60.2186) -> (76.6977, -60.0313)
  line L1023 (76.6977, -60.0313) -> (77.0083, -59.8964)
  line L1024 (77.0083, -59.8964) -> (77.0798, -59.8579)
  line L1025 (77.0798, -59.8579) -> (77.149, -59.8141)
  line L1026 (77.149, -59.8141) -> (77.2167, -59.7668)
  line L1027 (77.2167, -59.7668) -> (77.2831, -59.7166)
  line L1028 (77.2831, -59.7166) -> (77.3483, -59.6639)
  line L1029 (77.3483, -59.6639) -> (77.4124, -59.6088)
  line L1030 (77.4124, -59.6088) -> (77.4755, -59.5517)
  line L1031 (77.4755, -59.5517) -> (77.5376, -59.4925)
  line L1032 (77.5376, -59.4925) -> (77.5988, -59.4315)
  line L1033 (77.5988, -59.4315) -> (77.6591, -59.3687)
  line L1034 (77.6591, -59.3687) -> (77.7184, -59.3041)
  line L1035 (77.7184, -59.3041) -> (77.7769, -59.2378)
  line L1036 (77.7769, -59.2378) -> (77.7164, -59.1103)
  line L1037 (77.7164, -59.1103) -> (77.6543, -58.9836)
  line L1038 (77.6543, -58.9836) -> (77.5906, -58.8577)
  line L1039 (77.5906, -58.8577) -> (77.5025, -58.8633)
  line L1040 (77.5025, -58.8633) -> (77.415, -58.8707)
  line L1041 (77.415, -58.8707) -> (77.3285, -58.8798)
  line L1042 (77.3285, -58.8798) -> (77.2427, -58.8907)
  line L1043 (77.2427, -58.8907) -> (77.1579, -58.9036)
  line L1044 (77.1579, -58.9036) -> (77.0741, -58.9185)
  line L1045 (77.0741, -58.9185) -> (76.9913, -58.9354)
  line L1046 (76.9913, -58.9354) -> (76.9097, -58.9546)
  line L1047 (76.9097, -58.9546) -> (76.8294, -58.9763)
  line L1048 (76.8294, -58.9763) -> (76.7505, -59.0008)
  line L1049 (76.7505, -59.0008) -> (76.6735, -59.0286)
  line L1050 (76.6735, -59.0286) -> (76.5992, -59.0616)
  line L1051 (76.5992, -59.0616) -> (76.3023, -59.2244)
  line L1052 (76.3023, -59.2244) -> (76.2027, -59.0471)
  line L1053 (76.2027, -59.0471) -> (76.0995, -58.872)
  line L1054 (76.0995, -58.872) -> (75.9927, -58.699)
  line L1055 (75.9927, -58.699) -> (75.8823, -58.5283)
  line L1056 (75.8823, -58.5283) -> (76.1648, -58.3415)
  line L1057 (76.1648, -58.3415) -> (76.2285, -58.2911)
  line L1058 (76.2285, -58.2911) -> (76.289, -58.2359)
  line L1059 (76.289, -58.2359) -> (76.3474, -58.1776)
  line L1060 (76.3474, -58.1776) -> (76.4041, -58.1167)
  line L1061 (76.4041, -58.1167) -> (76.4591, -58.0534)
  line L1062 (76.4591, -58.0534) -> (76.5127, -57.9881)
  line L1063 (76.5127, -57.9881) -> (76.5649, -57.9209)
  line L1064 (76.5649, -57.9209) -> (76.6159, -57.8518)
  line L1065 (76.6159, -57.8518) -> (76.6655, -57.7811)
  line L1066 (76.6655, -57.7811) -> (76.714, -57.7087)
  line L1067 (76.714, -57.7087) -> (76.7612, -57.6348)
  line L1068 (76.7612, -57.6348) -> (76.8073, -57.5594)
  line L1069 (76.8073, -57.5594) -> (76.7256, -57.4444)
  line L1070 (76.7256, -57.4444) -> (76.6424, -57.3304)
  line L1071 (76.6424, -57.3304) -> (76.5579, -57.2174)
  line L1072 (76.5579, -57.2174) -> (76.472, -57.2383)
  line L1073 (76.472, -57.2383) -> (76.3872, -57.2607)
  line L1074 (76.3872, -57.2607) -> (76.3035, -57.2847)
  line L1075 (76.3035, -57.2847) -> (76.2209, -57.3104)
  line L1076 (76.2209, -57.3104) -> (76.1397, -57.3378)
  line L1077 (76.1397, -57.3378) -> (76.0597, -57.367)
  line L1078 (76.0597, -57.367) -> (75.9811, -57.398)
  line L1079 (75.9811, -57.398) -> (75.9041, -57.4311)
  line L1080 (75.9041, -57.4311) -> (75.8287, -57.4664)
  line L1081 (75.8287, -57.4664) -> (75.7553, -57.5042)
  line L1082 (75.7553, -57.5042) -> (75.6843, -57.545)
  line L1083 (75.6843, -57.545) -> (75.6169, -57.5903)
  line L1084 (75.6169, -57.5903) -> (75.3527, -57.8022)
  line L1085 (75.3527, -57.8022) -> (75.2239, -57.645)
  line L1086 (75.2239, -57.645) -> (75.0918, -57.4904)
  line L1087 (75.0918, -57.4904) -> (74.9566, -57.3386)
  line L1088 (74.9566, -57.3386) -> (74.8182, -57.1897)
  line L1089 (74.8182, -57.1897) -> (75.064, -56.9566)
  line L1090 (75.064, -56.9566) -> (75.118, -56.896)
  line L1091 (75.118, -56.896) -> (75.1681, -56.8311)
  line L1092 (75.1681, -56.8311) -> (75.2154, -56.7635)
  line L1093 (75.2154, -56.7635) -> (75.2606, -56.6937)
  line L1094 (75.2606, -56.6937) -> (75.3039, -56.6218)
  line L1095 (75.3039, -56.6218) -> (75.3453, -56.5482)
  line L1096 (75.3453, -56.5482) -> (75.3851, -56.4729)
  line L1097 (75.3851, -56.4729) -> (75.4232, -56.3961)
  line L1098 (75.4232, -56.3961) -> (75.4598, -56.3178)
  line L1099 (75.4598, -56.3178) -> (75.495, -56.2381)
  line L1100 (75.495, -56.2381) -> (75.5287, -56.1571)
  line L1101 (75.5287, -56.1571) -> (75.5609, -56.0749)
  line L1102 (75.5609, -56.0749) -> (75.4605, -55.9758)
  line L1103 (75.4605, -55.9758) -> (75.3588, -55.878)
  line L1104 (75.3588, -55.878) -> (75.2559, -55.7814)
  line L1105 (75.2559, -55.7814) -> (75.175, -55.8169)
  line L1106 (75.175, -55.8169) -> (75.0953, -55.8536)
  line L1107 (75.0953, -55.8536) -> (75.0171, -55.8918)
  line L1108 (75.0171, -55.8918) -> (74.9403, -55.9314)
  line L1109 (74.9403, -55.9314) -> (74.865, -55.9725)
  line L1110 (74.865, -55.9725) -> (74.7913, -56.0152)
  line L1111 (74.7913, -56.0152) -> (74.7193, -56.0594)
  line L1112 (74.7193, -56.0594) -> (74.6492, -56.1054)
  line L1113 (74.6492, -56.1054) -> (74.5811, -56.1532)
  line L1114 (74.5811, -56.1532) -> (74.5154, -56.2032)
  line L1115 (74.5154, -56.2032) -> (74.4526, -56.2557)
  line L1116 (74.4526, -56.2557) -> (74.394, -56.312)
  line L1117 (74.394, -56.312) -> (74.1706, -56.5666)
  line L1118 (74.1706, -56.5666) -> (74.0165, -56.4341)
  line L1119 (74.0165, -56.4341) -> (73.8596, -56.3048)
  line L1120 (73.8596, -56.3048) -> (73.7, -56.1788)
  line L1121 (73.7, -56.1788) -> (73.5379, -56.0562)
  line L1122 (73.5379, -56.0562) -> (73.7395, -55.784)
  line L1123 (73.7395, -55.784) -> (73.7821, -55.7149)
  line L1124 (73.7821, -55.7149) -> (73.8202, -55.6423)
  line L1125 (73.8202, -55.6423) -> (73.8551, -55.5675)
  line L1126 (73.8551, -55.5675) -> (73.8875, -55.4909)
  line L1127 (73.8875, -55.4909) -> (73.9176, -55.4126)
  line L1128 (73.9176, -55.4126) -> (73.9456, -55.3329)
  line L1129 (73.9456, -55.3329) -> (73.9717, -55.2519)
  line L1130 (73.9717, -55.2519) -> (73.9959, -55.1696)
  line L1131 (73.9959, -55.1696) -> (74.0184, -55.0861)
  line L1132 (74.0184, -55.0861) -> (74.0391, -55.0016)
  line L1133 (74.0391, -55.0016) -> (74.0582, -54.916)
  line L1134 (74.0582, -54.916) -> (74.0758, -54.8293)
  line L1135 (74.0758, -54.8293) -> (73.9596, -54.7492)
  line L1136 (73.9596, -54.7492) -> (73.8425, -54.6705)
  line L1137 (73.8425, -54.6705) -> (73.7244, -54.5933)
  line L1138 (73.7244, -54.5933) -> (73.6508, -54.6422)
  line L1139 (73.6508, -54.6422) -> (73.5788, -54.6923)
  line L1140 (73.5788, -54.6923) -> (73.5084, -54.7435)
  line L1141 (73.5084, -54.7435) -> (73.4396, -54.7959)
  line L1142 (73.4396, -54.7959) -> (73.3726, -54.8494)
  line L1143 (73.3726, -54.8494) -> (73.3074, -54.9042)
  line L1144 (73.3074, -54.9042) -> (73.2442, -54.9602)
  line L1145 (73.2442, -54.9602) -> (73.1831, -55.0177)
  line L1146 (73.1831, -55.0177) -> (73.1244, -55.0766)
  line L1147 (73.1244, -55.0766) -> (73.0684, -55.1373)
  line L1148 (73.0684, -55.1373) -> (73.0156, -55.1999)
  line L1149 (73.0156, -55.1999) -> (72.9677, -55.2655)
  line L1150 (72.9677, -55.2655) -> (72.792, -55.555)
  line L1151 (72.792, -55.555) -> (72.6171, -55.4513)
  line L1152 (72.6171, -55.4513) -> (72.4401, -55.3512)
  line L1153 (72.4401, -55.3512) -> (72.2612, -55.2548)
  line L1154 (72.2612, -55.2548) -> (72.0802, -55.1622)
  line L1155 (72.0802, -55.1622) -> (72.2314, -54.8591)
  line L1156 (72.2314, -54.8591) -> (72.2614, -54.7837)
  line L1157 (72.2614, -54.7837) -> (72.2863, -54.7056)
  line L1158 (72.2863, -54.7056) -> (72.3077, -54.6259)
  line L1159 (72.3077, -54.6259) -> (72.3263, -54.5448)
  line L1160 (72.3263, -54.5448) -> (72.3423, -54.4625)
  line L1161 (72.3423, -54.4625) -> (72.3561, -54.3791)
  line L1162 (72.3561, -54.3791) -> (72.3677, -54.2948)
  line L1163 (72.3677, -54.2948) -> (72.3773, -54.2096)
  line L1164 (72.3773, -54.2096) -> (72.3849, -54.1235)
  line L1165 (72.3849, -54.1235) -> (72.3907, -54.0366)
  line L1166 (72.3907, -54.0366) -> (72.3946, -53.9489)
  line L1167 (72.3946, -53.9489) -> (72.3968, -53.8606)
  line L1168 (72.3968, -53.8606) -> (72.2686, -53.8018)
  line L1169 (72.2686, -53.8018) -> (72.1396, -53.7447)
  line L1170 (72.1396, -53.7447) -> (72.0099, -53.6892)
  line L1171 (72.0099, -53.6892) -> (71.9459, -53.7501)
  line L1172 (71.9459, -53.7501) -> (71.8837, -53.812)
  line L1173 (71.8837, -53.812) -> (71.8232, -53.8746)
  line L1174 (71.8232, -53.8746) -> (71.7645, -53.9381)
  line L1175 (71.7645, -53.9381) -> (71.7078, -54.0025)
  line L1176 (71.7078, -54.0025) -> (71.6532, -54.0677)
  line L1177 (71.6532, -54.0677) -> (71.6007, -54.1339)
  line L1178 (71.6007, -54.1339) -> (71.5505, -54.2011)
  line L1179 (71.5505, -54.2011) -> (71.5029, -54.2694)
  line L1180 (71.5029, -54.2694) -> (71.4582, -54.3388)
  line L1181 (71.4582, -54.3388) -> (71.4171, -54.4096)
  line L1182 (71.4171, -54.4096) -> (71.3814, -54.4826)
  line L1183 (71.3814, -54.4826) -> (71.2586, -54.7982)
  line L1184 (71.2586, -54.7982) -> (71.0684, -54.7264)
  line L1185 (71.0684, -54.7264) -> (70.8767, -54.6586)
  line L1186 (70.8767, -54.6586) -> (70.6837, -54.5948)
  line L1187 (70.6837, -54.5948) -> (70.4894, -54.5349)
extrude "Extrude1''''" add sketch "Sketch1 (5)" along normal blind 2.5 separate body makes body 8 in component "CT dial wheel (tool body)"
ref_plane "WorkPlane2" through (0, 0, 43.4) normal (0, 0, 1) x (1, 0, 0) in component "CT dial wheel (tool body)"
sketch "Sketch2 (4)" plane through (0, 0, 43.4) normal (0, 0, 1) x (1, 0, 0) in component "CT dial wheel (tool body)"
  circle A0 centre (67.7, -63.94) radius 1.6
extrude "Extrude2'''" cut sketch "Sketch2 (4)" along normal blind 2.5 bodies 8 in component "CT dial wheel (tool body)"
component "CT sprocket pinion (tool body)" placed x (1, 0, 0) y (0, 1, 0) z (0, 0, 1) at (0, 0, 0)
component "CT idler 1" placed x (1, 0, 0) y (0, 1, 0) z (0, 0, 1) at (0, 0, 0)
component "CT idler 2" placed x (1, 0, 0) y (0, 1, 0) z (0, 0, 1) at (0, 0, 0)
component "CT idler 3" placed x (1, 0, 0) y (0, 1, 0) z (0, 0, 1) at (0, 0, 0)
component "CT dial wheel (tool body)" placed x (1, 0, 0) y (0, 1, 0) z (0, 0, 1) at (0, 0, 0)
equation "ct_module = 0.6 mm" comment "Counter train: gear module"
equation "ct_pressure_angle = 20.0 deg" comment "Counter train: pressure angle"
equation "ct_pinion_teeth = 12" comment "Counter train: teeth on every pinion"
equation "ct_wheel1_teeth = 32" comment "Counter train: idler 1 wheel (meshes sprocket pinion)"
equation "ct_wheel2_teeth = 30" comment "Counter train: idler 2 wheel"
equation "ct_wheel3_teeth = 30" comment "Counter train: idler 3 wheel"
equation "ct_wheel4_teeth = 36" comment "Counter train: dial wheel"
equation "ct_thinning = 0.1 mm" comment "Counter train: tooth thinning per gear (backlash share)"
equation "ct_pinion_shift = 0.4" comment "Counter train: pinion profile shift x (wheels get -x)"
equation "ct_pinion_tip_reduction = 0.1 mm" comment "Counter train: pinion tip shave (radial)"
equation "ct_wheel_tip_reduction = 0.04 mm" comment "Counter train: wheel tip shave (radial)"
equation "ct_sprocket_x = 73.2 mm" comment "Counter train: sprocket axis X (fixed)"
equation "ct_sprocket_y = -45.21 mm" comment "Counter train: sprocket axis Y (fixed)"
equation "ct_dial_x = 67.7 mm" comment "Counter train: dial axis X (fixed)"
equation "ct_dial_y = -63.94 mm" comment "Counter train: dial axis Y (fixed)"
equation "ct_idler1_angle = -90.74 deg" comment "Counter train: direction sprocket -> idler 1"
equation "ct_idler2_angle = -164.0 deg" comment "Counter train: direction idler 1 -> idler 2"
equation "ct_idler3_elbow = 1" comment "Counter train: idler 3 solution, 1 or -1"
equation "ct_pinion0_z0 = 36.8 mm" comment "Counter train: sprocket pinion underside"
equation "ct_pinion0_z1 = 40.8 mm" comment "Counter train: sprocket pinion top"
equation "ct_wheel1_z0 = 36.8 mm" comment "Counter train: idler 1 wheel underside"
equation "ct_wheel1_z1 = 38.5 mm" comment "Counter train: idler 1 wheel top"
equation "ct_wheel2_z0 = 39.0 mm" comment "Counter train: idler 2 wheel underside"
equation "ct_wheel2_z1 = 40.8 mm" comment "Counter train: idler 2 wheel top"
equation "ct_wheel3_z0 = 41.2 mm" comment "Counter train: idler 3 wheel underside"
equation "ct_wheel3_z1 = 43.0 mm" comment "Counter train: idler 3 wheel top"
equation "ct_wheel4_z0 = 43.4 mm" comment "Counter train: dial wheel underside"
equation "ct_wheel4_z1 = 45.9 mm" comment "Counter train: dial wheel top"
equation "ct_pinion1_z1 = 40.8 mm" comment "Counter train: idler 1 pinion top (starts at its wheel top)"
equation "ct_pinion2_z1 = 43.0 mm" comment "Counter train: idler 2 pinion top (starts at its wheel top)"
equation "ct_pinion3_z1 = 45.4 mm" comment "Counter train: idler 3 pinion top (starts at its wheel top)"
equation "ct_pinion_phase = 15.0 deg" comment "Counter train: sprocket pinion tooth phase (others follow)"
equation "ct_clearance = 0.3 mm" comment "Counter train: minimum radial gap to non-meshing parts"
equation "ct_axial_clearance = 0.3 mm" comment "Counter train: minimum axial gap between stacked gears"
equation "ct_bore1 = 4.2 mm" comment "Counter train: idler 1 bore below the step"
equation "ct_bore1_upper = 3.4 mm" comment "Counter train: idler 1 bore above the step"
equation "ct_bore1_step_z = 38.8 mm" comment "Counter train: idler 1 bore step height"
equation "ct_bore2 = 3.4 mm" comment "Counter train: idler 2 bore below the step"
equation "ct_bore2_upper = 3.4 mm" comment "Counter train: idler 2 bore above the step"
equation "ct_bore2_step_z = 39.0 mm" comment "Counter train: idler 2 bore step height"
equation "ct_bore3 = 3.4 mm" comment "Counter train: idler 3 bore below the step"
equation "ct_bore3_upper = 3.4 mm" comment "Counter train: idler 3 bore above the step"
equation "ct_bore3_step_z = 41.2 mm" comment "Counter train: idler 3 bore step height"
equation "ct_bore4 = 3.2 mm" comment "Counter train: dial wheel bore below the step"
equation "ct_bore4_upper = 3.2 mm" comment "Counter train: dial wheel bore above the step"
equation "ct_bore4_step_z = 43.4 mm" comment "Counter train: dial wheel bore step height"
named bodies: "CT sprocket pinion (tool body)", "CT idler 1", "CT idler 1 pinion", "CT idler 2", "CT idler 2 pinion", "CT idler 3", "CT idler 3 pinion", "CT dial wheel (tool body)"
